Autodesk Inventor part; units mm, degrees
(part 2 of 2)
  line L438 (-36.1364, 2.6314) -> (-36.1459, 2.5251) construction
  line L439 (-36.1459, 2.5251) -> (-36.2475, 2.422) construction
  line L440 (-36.2475, 2.422) -> (-36.3751, 2.4459) construction
  line L441 (-36.3751, 2.4459) -> (-36.4459, 2.4614) construction
  spline S18 degree 3 poles (-38.8557, 2.1969) (-38.8572, 2.1987) (-38.8752, 2.2211) (-38.9092, 2.2645) (-38.9608, 2.3377) (-39.0083, 2.4172) (-39.0608, 2.5183) (-39.1072, 2.6209) (-39.1463, 2.7307) (-39.1715, 2.82) (-39.1895, 2.91) (-39.201, 2.9839) (-39.2117, 3.0528) (-39.2228, 3.1467) (-39.2255, 3.2598) (-39.2208, 3.3682) (-39.215, 3.4693) (-39.2042, 3.5799) (-39.184, 3.7003) (-39.135, 3.8891) (-39.034, 4.1141) (-38.8742, 4.3089) (-38.7335, 4.4249) (-38.62, 4.4967) (-38.5019, 4.5521) (-38.3842, 4.5944) (-38.2605, 4.6297) (-38.1226, 4.6549) (-37.9886, 4.6632) (-37.8833, 4.6627) (-37.7903, 4.6606) (-37.6909, 4.6547) (-37.5837, 4.6412) (-37.4418, 4.6164) (-37.3105, 4.5895) (-37.1813, 4.5608) (-37.0882, 4.538) (-36.9992, 4.5129) (-36.8769, 4.476) (-36.7073, 4.4231) (-36.5, 4.351) (-36.3059, 4.2743) (-36.1511, 4.2074) (-36.0218, 4.1447) (-35.903, 4.0832) (-35.7462, 3.9967) (-35.5515, 3.8647) (-35.3733, 3.7141) (-35.2209, 3.5517) (-35.1421, 3.4422) (-35.1062, 3.3821) knots 0 0 0 0 0.001093 0.013473 0.025854 0.039399 0.052944 0.078386 0.091133 0.103881 0.117308 0.130735 0.141579 0.152424 0.170959 0.189495 0.205461 0.221427 0.240479 0.259531 0.305769 0.343024 0.361055 0.379086 0.396915 0.414744 0.434745 0.454745 0.473468 0.492192 0.505844 0.519497 0.537166 0.554835 0.590157 0.606148 0.622138 0.636609 0.651081 0.687747 0.728505 0.761398 0.793268 0.812623 0.831977 0.860868 0.899522 0.942063 0.970647 1 1 1 1
  line L442 (-38.8557, 2.1969) -> (-38.8572, 2.1987) construction
  line L443 (-38.8572, 2.1987) -> (-38.8752, 2.2211) construction
  line L444 (-38.8752, 2.2211) -> (-38.9092, 2.2645) construction
  line L445 (-38.9092, 2.2645) -> (-38.9608, 2.3377) construction
  line L446 (-38.9608, 2.3377) -> (-39.0083, 2.4172) construction
  line L447 (-39.0083, 2.4172) -> (-39.0608, 2.5183) construction
  line L448 (-39.0608, 2.5183) -> (-39.1072, 2.6209) construction
  line L449 (-39.1072, 2.6209) -> (-39.1463, 2.7307) construction
  line L450 (-39.1463, 2.7307) -> (-39.1715, 2.82) construction
  line L451 (-39.1715, 2.82) -> (-39.1895, 2.91) construction
  line L452 (-39.1895, 2.91) -> (-39.201, 2.9839) construction
  line L453 (-39.201, 2.9839) -> (-39.2117, 3.0528) construction
  line L454 (-39.2117, 3.0528) -> (-39.2228, 3.1467) construction
  line L455 (-39.2228, 3.1467) -> (-39.2255, 3.2598) construction
  line L456 (-39.2255, 3.2598) -> (-39.2208, 3.3682) construction
  line L457 (-39.2208, 3.3682) -> (-39.215, 3.4693) construction
  line L458 (-39.215, 3.4693) -> (-39.2042, 3.5799) construction
  line L459 (-39.2042, 3.5799) -> (-39.184, 3.7003) construction
  line L460 (-39.184, 3.7003) -> (-39.135, 3.8891) construction
  line L461 (-39.135, 3.8891) -> (-39.034, 4.1141) construction
  line L462 (-39.034, 4.1141) -> (-38.8742, 4.3089) construction
  line L463 (-38.8742, 4.3089) -> (-38.7335, 4.4249) construction
  line L464 (-38.7335, 4.4249) -> (-38.62, 4.4967) construction
  line L465 (-38.62, 4.4967) -> (-38.5019, 4.5521) construction
  line L466 (-38.5019, 4.5521) -> (-38.3842, 4.5944) construction
  line L467 (-38.3842, 4.5944) -> (-38.2605, 4.6297) construction
  line L468 (-38.2605, 4.6297) -> (-38.1226, 4.6549) construction
  line L469 (-38.1226, 4.6549) -> (-37.9886, 4.6632) construction
  line L470 (-37.9886, 4.6632) -> (-37.8833, 4.6627) construction
  line L471 (-37.8833, 4.6627) -> (-37.7903, 4.6606) construction
  line L472 (-37.7903, 4.6606) -> (-37.6909, 4.6547) construction
  line L473 (-37.6909, 4.6547) -> (-37.5837, 4.6412) construction
  line L474 (-37.5837, 4.6412) -> (-37.4418, 4.6164) construction
  line L475 (-37.4418, 4.6164) -> (-37.3105, 4.5895) construction
  line L476 (-37.3105, 4.5895) -> (-37.1813, 4.5608) construction
  line L477 (-37.1813, 4.5608) -> (-37.0882, 4.538) construction
  line L478 (-37.0882, 4.538) -> (-36.9992, 4.5129) construction
  line L479 (-36.9992, 4.5129) -> (-36.8769, 4.476) construction
  line L480 (-36.8769, 4.476) -> (-36.7073, 4.4231) construction
  line L481 (-36.7073, 4.4231) -> (-36.5, 4.351) construction
  line L482 (-36.5, 4.351) -> (-36.3059, 4.2743) construction
  line L483 (-36.3059, 4.2743) -> (-36.1511, 4.2074) construction
  line L484 (-36.1511, 4.2074) -> (-36.0218, 4.1447) construction
  line L485 (-36.0218, 4.1447) -> (-35.903, 4.0832) construction
  line L486 (-35.903, 4.0832) -> (-35.7462, 3.9967) construction
  line L487 (-35.7462, 3.9967) -> (-35.5515, 3.8647) construction
  line L488 (-35.5515, 3.8647) -> (-35.3733, 3.7141) construction
  line L489 (-35.3733, 3.7141) -> (-35.2209, 3.5517) construction
  line L490 (-35.2209, 3.5517) -> (-35.1421, 3.4422) construction
  line L491 (-35.1421, 3.4422) -> (-35.1062, 3.3821) construction
  spline S19 degree 3 poles (-35.3209, 3.254) (-35.3774, 3.3487) (-35.5015, 3.4947) (-35.7033, 3.6655) (-35.8763, 3.7828) (-36.0526, 3.8802) (-36.221, 3.9652) (-36.4011, 4.0431) (-36.5871, 4.1166) (-36.7846, 4.1853) (-36.9771, 4.2453) (-37.1543, 4.2983) (-37.3323, 4.3387) (-37.5228, 4.3778) (-37.7065, 4.4078) (-37.8961, 4.4137) (-38.0956, 4.4123) (-38.3052, 4.3609) (-38.5029, 4.2823) (-38.6723, 4.1597) (-38.8176, 3.9829) (-38.9138, 3.7703) (-38.9587, 3.5534) (-38.9723, 3.3509) (-38.9778, 3.1783) (-38.9534, 3.0176) (-38.9313, 2.8789) (-38.8857, 2.7381) (-38.8248, 2.6032) (-38.7544, 2.4743) (-38.6401, 2.3235) (-38.5475, 2.2212) (-38.4765, 2.1644) knots 0 0 0 0 0.055351 0.095994 0.132923 0.160524 0.197506 0.227953 0.259379 0.298318 0.333348 0.360999 0.391552 0.425298 0.459059 0.485146 0.520921 0.559137 0.593204 0.627656 0.663248 0.707423 0.743827 0.774334 0.80975 0.830472 0.856127 0.880484 0.904791 0.930672 0.954328 1 1 1 1
  line L492 (-35.3209, 3.254) -> (-35.3774, 3.3487) construction
  line L493 (-35.3774, 3.3487) -> (-35.5015, 3.4947) construction
  line L494 (-35.5015, 3.4947) -> (-35.7033, 3.6655) construction
  line L495 (-35.7033, 3.6655) -> (-35.8763, 3.7828) construction
  line L496 (-35.8763, 3.7828) -> (-36.0526, 3.8802) construction
  line L497 (-36.0526, 3.8802) -> (-36.221, 3.9652) construction
  line L498 (-36.221, 3.9652) -> (-36.4011, 4.0431) construction
  line L499 (-36.4011, 4.0431) -> (-36.5871, 4.1166) construction
  line L500 (-36.5871, 4.1166) -> (-36.7846, 4.1853) construction
  line L501 (-36.7846, 4.1853) -> (-36.9771, 4.2453) construction
  line L502 (-36.9771, 4.2453) -> (-37.1543, 4.2983) construction
  line L503 (-37.1543, 4.2983) -> (-37.3323, 4.3387) construction
  line L504 (-37.3323, 4.3387) -> (-37.5228, 4.3778) construction
  line L505 (-37.5228, 4.3778) -> (-37.7065, 4.4078) construction
  line L506 (-37.7065, 4.4078) -> (-37.8961, 4.4137) construction
  line L507 (-37.8961, 4.4137) -> (-38.0956, 4.4123) construction
  line L508 (-38.0956, 4.4123) -> (-38.3052, 4.3609) construction
  line L509 (-38.3052, 4.3609) -> (-38.5029, 4.2823) construction
  line L510 (-38.5029, 4.2823) -> (-38.6723, 4.1597) construction
  line L511 (-38.6723, 4.1597) -> (-38.8176, 3.9829) construction
  line L512 (-38.8176, 3.9829) -> (-38.9138, 3.7703) construction
  line L513 (-38.9138, 3.7703) -> (-38.9587, 3.5534) construction
  line L514 (-38.9587, 3.5534) -> (-38.9723, 3.3509) construction
  line L515 (-38.9723, 3.3509) -> (-38.9778, 3.1783) construction
  line L516 (-38.9778, 3.1783) -> (-38.9534, 3.0176) construction
  line L517 (-38.9534, 3.0176) -> (-38.9313, 2.8789) construction
  line L518 (-38.9313, 2.8789) -> (-38.8857, 2.7381) construction
  line L519 (-38.8857, 2.7381) -> (-38.8248, 2.6032) construction
  line L520 (-38.8248, 2.6032) -> (-38.7544, 2.4743) construction
  line L521 (-38.7544, 2.4743) -> (-38.6401, 2.3235) construction
  line L522 (-38.6401, 2.3235) -> (-38.5475, 2.2212) construction
  line L523 (-38.5475, 2.2212) -> (-38.4765, 2.1644) construction
  spline S20 degree 3 poles (-35.1062, 3.3821) (-35.0856, 3.3476) (-35.0436, 3.2753) (-34.9846, 3.1561) (-34.9385, 3.0325) (-34.8891, 2.8556) (-34.8509, 2.5961) (-34.8504, 2.2727) (-34.9129, 1.9367) (-35.0543, 1.6251) (-35.2047, 1.4458) (-35.3027, 1.3649) knots 0 0 0 0 0.062149 0.124299 0.18074 0.237181 0.376996 0.554667 0.704453 0.841631 1 1 1 1
  line L524 (-35.1062, 3.3821) -> (-35.0856, 3.3476) construction
  line L525 (-35.0856, 3.3476) -> (-35.0436, 3.2753) construction
  line L526 (-35.0436, 3.2753) -> (-34.9846, 3.1561) construction
  line L527 (-34.9846, 3.1561) -> (-34.9385, 3.0325) construction
  line L528 (-34.9385, 3.0325) -> (-34.8891, 2.8556) construction
  line L529 (-34.8891, 2.8556) -> (-34.8509, 2.5961) construction
  line L530 (-34.8509, 2.5961) -> (-34.8504, 2.2727) construction
  line L531 (-34.8504, 2.2727) -> (-34.9129, 1.9367) construction
  line L532 (-34.9129, 1.9367) -> (-35.0543, 1.6251) construction
  line L533 (-35.0543, 1.6251) -> (-35.2047, 1.4458) construction
  line L534 (-35.2047, 1.4458) -> (-35.3027, 1.3649) construction
  spline S21 degree 3 poles (-35.7186, 1.4187) (-35.5281, 1.4749) (-35.3089, 1.6711) (-35.1543, 2.0105) (-35.1011, 2.292) (-35.1012, 2.5793) (-35.14, 2.8406) (-35.2106, 3.0616) (-35.282, 3.1887) (-35.3209, 3.254) knots 0 0 0 0 0.273796 0.392161 0.521403 0.674708 0.795348 0.892748 1 1 1 1
  line L535 (-35.7186, 1.4187) -> (-35.5281, 1.4749) construction
  line L536 (-35.5281, 1.4749) -> (-35.3089, 1.6711) construction
  line L537 (-35.3089, 1.6711) -> (-35.1543, 2.0105) construction
  line L538 (-35.1543, 2.0105) -> (-35.1011, 2.292) construction
  line L539 (-35.1011, 2.292) -> (-35.1012, 2.5793) construction
  line L540 (-35.1012, 2.5793) -> (-35.14, 2.8406) construction
  line L541 (-35.14, 2.8406) -> (-35.2106, 3.0616) construction
  line L542 (-35.2106, 3.0616) -> (-35.282, 3.1887) construction
  line L543 (-35.282, 3.1887) -> (-35.3209, 3.254) construction
  spline S22 degree 3 poles (-35.1034, -2.5702) (-35.1001, -2.5752) (-35.0478, -2.6552) (-34.986, -2.7822) (-34.9281, -2.9499) (-34.8921, -3.0945) (-34.8696, -3.2455) (-34.8592, -3.3899) (-34.856, -3.5301) (-34.8648, -3.6828) (-34.895, -3.8447) (-34.9467, -4.0029) (-35.0178, -4.1531) (-35.1217, -4.3066) (-35.267, -4.4488) (-35.4359, -4.552) (-35.598, -4.6097) (-35.7882, -4.649) (-36.0245, -4.6565) (-36.338, -4.6162) (-36.6524, -4.5374) (-36.8714, -4.4666) (-36.9719, -4.4336) knots 0 0 0 0 0.00444 0.070664 0.108166 0.145668 0.1883 0.230932 0.268421 0.305909 0.348993 0.392077 0.432213 0.472349 0.522082 0.571814 0.60605 0.640285 0.714979 0.789672 0.901222 1 1 1 1
  line L544 (-35.1034, -2.5702) -> (-35.1001, -2.5752) construction
  line L545 (-35.1001, -2.5752) -> (-35.0478, -2.6552) construction
  line L546 (-35.0478, -2.6552) -> (-34.986, -2.7822) construction
  line L547 (-34.986, -2.7822) -> (-34.9281, -2.9499) construction
  line L548 (-34.9281, -2.9499) -> (-34.8921, -3.0945) construction
  line L549 (-34.8921, -3.0945) -> (-34.8696, -3.2455) construction
  line L550 (-34.8696, -3.2455) -> (-34.8592, -3.3899) construction
  line L551 (-34.8592, -3.3899) -> (-34.856, -3.5301) construction
  line L552 (-34.856, -3.5301) -> (-34.8648, -3.6828) construction
  line L553 (-34.8648, -3.6828) -> (-34.895, -3.8447) construction
  line L554 (-34.895, -3.8447) -> (-34.9467, -4.0029) construction
  line L555 (-34.9467, -4.0029) -> (-35.0178, -4.1531) construction
  line L556 (-35.0178, -4.1531) -> (-35.1217, -4.3066) construction
  line L557 (-35.1217, -4.3066) -> (-35.267, -4.4488) construction
  line L558 (-35.267, -4.4488) -> (-35.4359, -4.552) construction
  line L559 (-35.4359, -4.552) -> (-35.598, -4.6097) construction
  line L560 (-35.598, -4.6097) -> (-35.7882, -4.649) construction
  line L561 (-35.7882, -4.649) -> (-36.0245, -4.6565) construction
  line L562 (-36.0245, -4.6565) -> (-36.338, -4.6162) construction
  line L563 (-36.338, -4.6162) -> (-36.6524, -4.5374) construction
  line L564 (-36.6524, -4.5374) -> (-36.8714, -4.4666) construction
  line L565 (-36.8714, -4.4666) -> (-36.9719, -4.4336) construction
  spline S23 degree 3 poles (-36.9719, -4.4336) (-37.0123, -4.4203) (-37.0897, -4.3922) (-37.2189, -4.342) (-37.3714, -4.2863) (-37.5356, -4.2233) (-37.6712, -4.1641) (-37.8012, -4.1048) (-37.9577, -4.0339) (-38.1361, -3.9493) (-38.3019, -3.864) (-38.4383, -3.7917) (-38.5691, -3.7231) (-38.6924, -3.6501) (-38.8071, -3.5657) (-38.9238, -3.4587) (-39.0391, -3.3162) (-39.129, -3.1482) (-39.1807, -2.9867) (-39.2052, -2.8557) (-39.217, -2.7336) (-39.2183, -2.6183) (-39.2094, -2.5046) (-39.1927, -2.3995) (-39.1684, -2.2913) (-39.1263, -2.1755) (-39.0633, -2.0679) (-38.991, -1.9827) (-38.9362, -1.9368) (-38.9114, -1.9187) knots 0 0 0 0 0.033633 0.067267 0.12497 0.182674 0.216203 0.249732 0.309838 0.369945 0.420395 0.470846 0.5098 0.548753 0.581089 0.613424 0.660377 0.707331 0.741496 0.77566 0.80376 0.83186 0.859174 0.886489 0.912352 0.938215 0.960595 0.982975 1 1 1 1
  line L566 (-36.9719, -4.4336) -> (-37.0123, -4.4203) construction
  line L567 (-37.0123, -4.4203) -> (-37.0897, -4.3922) construction
  line L568 (-37.0897, -4.3922) -> (-37.2189, -4.342) construction
  line L569 (-37.2189, -4.342) -> (-37.3714, -4.2863) construction
  line L570 (-37.3714, -4.2863) -> (-37.5356, -4.2233) construction
  line L571 (-37.5356, -4.2233) -> (-37.6712, -4.1641) construction
  line L572 (-37.6712, -4.1641) -> (-37.8012, -4.1048) construction
  line L573 (-37.8012, -4.1048) -> (-37.9577, -4.0339) construction
  line L574 (-37.9577, -4.0339) -> (-38.1361, -3.9493) construction
  line L575 (-38.1361, -3.9493) -> (-38.3019, -3.864) construction
  line L576 (-38.3019, -3.864) -> (-38.4383, -3.7917) construction
  line L577 (-38.4383, -3.7917) -> (-38.5691, -3.7231) construction
  line L578 (-38.5691, -3.7231) -> (-38.6924, -3.6501) construction
  line L579 (-38.6924, -3.6501) -> (-38.8071, -3.5657) construction
  line L580 (-38.8071, -3.5657) -> (-38.9238, -3.4587) construction
  line L581 (-38.9238, -3.4587) -> (-39.0391, -3.3162) construction
  line L582 (-39.0391, -3.3162) -> (-39.129, -3.1482) construction
  line L583 (-39.129, -3.1482) -> (-39.1807, -2.9867) construction
  line L584 (-39.1807, -2.9867) -> (-39.2052, -2.8557) construction
  line L585 (-39.2052, -2.8557) -> (-39.217, -2.7336) construction
  line L586 (-39.217, -2.7336) -> (-39.2183, -2.6183) construction
  line L587 (-39.2183, -2.6183) -> (-39.2094, -2.5046) construction
  line L588 (-39.2094, -2.5046) -> (-39.1927, -2.3995) construction
  line L589 (-39.1927, -2.3995) -> (-39.1684, -2.2913) construction
  line L590 (-39.1684, -2.2913) -> (-39.1263, -2.1755) construction
  line L591 (-39.1263, -2.1755) -> (-39.0633, -2.0679) construction
  line L592 (-39.0633, -2.0679) -> (-38.991, -1.9827) construction
  line L593 (-38.991, -1.9827) -> (-38.9362, -1.9368) construction
  line L594 (-38.9362, -1.9368) -> (-38.9114, -1.9187) construction
  spline S24 degree 3 poles (-38.9114, -1.9187) (-38.9251, -1.9011) (-38.9697, -1.8403) (-39.0351, -1.7307) (-39.0942, -1.6025) (-39.1398, -1.4803) (-39.181, -1.3363) (-39.2151, -1.1313) (-39.2281, -0.9209) (-39.2377, -0.6906) (-39.226, -0.4881) (-39.1858, -0.3064) (-39.1385, -0.1725) (-39.0783, -0.0531) (-39.0252, 0.0316) (-38.9882, 0.0842) (-38.973, 0.104) knots 0 0 0 0 0.029625 0.099401 0.169177 0.226396 0.283615 0.373252 0.518061 0.616606 0.732557 0.796641 0.860726 0.914778 0.96883 1 1 1 1
  line L595 (-38.9114, -1.9187) -> (-38.9251, -1.9011) construction
  line L596 (-38.9251, -1.9011) -> (-38.9697, -1.8403) construction
  line L597 (-38.9697, -1.8403) -> (-39.0351, -1.7307) construction
  line L598 (-39.0351, -1.7307) -> (-39.0942, -1.6025) construction
  line L599 (-39.0942, -1.6025) -> (-39.1398, -1.4803) construction
  line L600 (-39.1398, -1.4803) -> (-39.181, -1.3363) construction
  line L601 (-39.181, -1.3363) -> (-39.2151, -1.1313) construction
  line L602 (-39.2151, -1.1313) -> (-39.2281, -0.9209) construction
  line L603 (-39.2281, -0.9209) -> (-39.2377, -0.6906) construction
  line L604 (-39.2377, -0.6906) -> (-39.226, -0.4881) construction
  line L605 (-39.226, -0.4881) -> (-39.1858, -0.3064) construction
  line L606 (-39.1858, -0.3064) -> (-39.1385, -0.1725) construction
  line L607 (-39.1385, -0.1725) -> (-39.0783, -0.0531) construction
  line L608 (-39.0783, -0.0531) -> (-39.0252, 0.0316) construction
  line L609 (-39.0252, 0.0316) -> (-38.9882, 0.0842) construction
  line L610 (-38.9882, 0.0842) -> (-38.973, 0.104) construction
  spline S25 degree 3 poles (-35.137, -0.7452) (-35.1273, -0.7589) (-35.0841, -0.8224) (-35.0167, -0.9412) (-34.9453, -1.1152) (-34.8975, -1.2995) (-34.8655, -1.5015) (-34.842, -1.7306) (-34.8544, -1.977) (-34.9084, -2.186) (-34.9802, -2.3655) (-35.0495, -2.4912) (-35.0989, -2.5638) (-35.1034, -2.5702) knots 0 0 0 0 0.025339 0.116179 0.207018 0.309076 0.411134 0.550932 0.69073 0.778469 0.866209 0.988083 1 1 1 1
  line L611 (-35.137, -0.7452) -> (-35.1273, -0.7589) construction
  line L612 (-35.1273, -0.7589) -> (-35.0841, -0.8224) construction
  line L613 (-35.0841, -0.8224) -> (-35.0167, -0.9412) construction
  line L614 (-35.0167, -0.9412) -> (-34.9453, -1.1152) construction
  line L615 (-34.9453, -1.1152) -> (-34.8975, -1.2995) construction
  line L616 (-34.8975, -1.2995) -> (-34.8655, -1.5015) construction
  line L617 (-34.8655, -1.5015) -> (-34.842, -1.7306) construction
  line L618 (-34.842, -1.7306) -> (-34.8544, -1.977) construction
  line L619 (-34.8544, -1.977) -> (-34.9084, -2.186) construction
  line L620 (-34.9084, -2.186) -> (-34.9802, -2.3655) construction
  line L621 (-34.9802, -2.3655) -> (-35.0495, -2.4912) construction
  line L622 (-35.0495, -2.4912) -> (-35.0989, -2.5638) construction
  line L623 (-35.0989, -2.5638) -> (-35.1034, -2.5702) construction
  arc A2 (-37.8544, -1.1308) -> (-37.4616, -1.3224) centre (-36.4977, 1.1532) ccw
  arc A3 (-36.7641, -1.5741) -> (-36.2828, -1.7225) centre (-35.1742, 2.7263) ccw
  spline S26 degree 3 poles (-36.7641, -1.5741) (-36.7505, -1.4891) (-36.7247, -1.3264) (-36.7301, -1.0707) (-36.8177, -0.8355) (-37.0007, -0.7186) (-37.1591, -0.6557) (-37.3343, -0.6531) (-37.4608, -0.8025) (-37.4863, -1.0375) (-37.4849, -1.2137) (-37.4616, -1.3224) knots 0.000002 0.000002 0.000002 0.000002 0.130512 0.248338 0.387441 0.486956 0.566128 0.647917 0.731171 0.833817 0.999993 0.999993 0.999993 0.999993
  line L624 (-36.7641, -1.5741) -> (-36.7505, -1.4891) construction
  line L625 (-36.7505, -1.4891) -> (-36.7247, -1.3264) construction
  line L626 (-36.7247, -1.3264) -> (-36.7301, -1.0707) construction
  line L627 (-36.7301, -1.0707) -> (-36.8177, -0.8355) construction
  line L628 (-36.8177, -0.8355) -> (-37.0007, -0.7186) construction
  line L629 (-37.0007, -0.7186) -> (-37.1591, -0.6557) construction
  line L630 (-37.1591, -0.6557) -> (-37.3343, -0.6531) construction
  line L631 (-37.3343, -0.6531) -> (-37.4608, -0.8025) construction
  line L632 (-37.4608, -0.8025) -> (-37.4863, -1.0375) construction
  line L633 (-37.4863, -1.0375) -> (-37.4849, -1.2137) construction
  line L634 (-37.4849, -1.2137) -> (-37.4616, -1.3224) construction
  spline S27 degree 3 poles (-35.4263, -2.5707) (-35.3321, -2.4741) (-35.2054, -2.2811) (-35.0814, -1.9154) (-35.1051, -1.552) (-35.1862, -1.1164) (-35.3442, -0.8602) (-35.473, -0.7347) knots 0 0 0 0 0.199784 0.341442 0.567149 0.731925 1 1 1 1
  line L635 (-35.4263, -2.5707) -> (-35.3321, -2.4741) construction
  line L636 (-35.3321, -2.4741) -> (-35.2054, -2.2811) construction
  line L637 (-35.2054, -2.2811) -> (-35.0814, -1.9154) construction
  line L638 (-35.0814, -1.9154) -> (-35.1051, -1.552) construction
  line L639 (-35.1051, -1.552) -> (-35.1862, -1.1164) construction
  line L640 (-35.1862, -1.1164) -> (-35.3442, -0.8602) construction
  line L641 (-35.3442, -0.8602) -> (-35.473, -0.7347) construction
  spline S28 degree 3 poles (-37.8544, -1.1308) (-37.8536, -0.9801) (-37.8499, -0.742) (-37.9125, -0.4332) (-38.0504, -0.2331) (-38.2518, -0.153) (-38.4786, -0.1595) (-38.6195, -0.3388) (-38.6813, -0.5514) (-38.6938, -0.7925) (-38.677, -1.0533) (-38.6261, -1.3179) (-38.5012, -1.5537) (-38.3084, -1.7405) (-38.0832, -1.8914) (-37.839, -2.0089) (-37.5863, -2.1154) (-37.3337, -2.2319) (-37.0665, -2.3111) (-36.8068, -2.3986) (-36.5292, -2.458) (-36.2438, -2.5065) (-35.9696, -2.5082) (-35.7113, -2.4196) (-35.5214, -2.2369) (-35.4217, -1.9412) (-35.3888, -1.645) (-35.4563, -1.3237) (-35.5661, -1.0472) (-35.7908, -0.8404) (-36.0487, -0.7938) (-36.2934, -0.8932) (-36.3899, -1.2666) (-36.3184, -1.5315) (-36.2828, -1.7225) knots 0.000002 0.000002 0.000002 0.000002 0.050812 0.079978 0.105051 0.128715 0.150613 0.176165 0.198359 0.225349 0.256757 0.286428 0.315385 0.345015 0.375912 0.406383 0.43613 0.468337 0.499902 0.529857 0.5606 0.595385 0.627424 0.651669 0.685878 0.711437 0.755573 0.784369 0.821416 0.854265 0.882212 0.905839 0.935385 1 1 1 1
  line L642 (-37.8544, -1.1308) -> (-37.8536, -0.9801) construction
  line L643 (-37.8536, -0.9801) -> (-37.8499, -0.742) construction
  line L644 (-37.8499, -0.742) -> (-37.9125, -0.4332) construction
  line L645 (-37.9125, -0.4332) -> (-38.0504, -0.2331) construction
  line L646 (-38.0504, -0.2331) -> (-38.2518, -0.153) construction
  line L647 (-38.2518, -0.153) -> (-38.4786, -0.1595) construction
  line L648 (-38.4786, -0.1595) -> (-38.6195, -0.3388) construction
  line L649 (-38.6195, -0.3388) -> (-38.6813, -0.5514) construction
  line L650 (-38.6813, -0.5514) -> (-38.6938, -0.7925) construction
  line L651 (-38.6938, -0.7925) -> (-38.677, -1.0533) construction
  line L652 (-38.677, -1.0533) -> (-38.6261, -1.3179) construction
  line L653 (-38.6261, -1.3179) -> (-38.5012, -1.5537) construction
  line L654 (-38.5012, -1.5537) -> (-38.3084, -1.7405) construction
  line L655 (-38.3084, -1.7405) -> (-38.0832, -1.8914) construction
  line L656 (-38.0832, -1.8914) -> (-37.839, -2.0089) construction
  line L657 (-37.839, -2.0089) -> (-37.5863, -2.1154) construction
  line L658 (-37.5863, -2.1154) -> (-37.3337, -2.2319) construction
  line L659 (-37.3337, -2.2319) -> (-37.0665, -2.3111) construction
  line L660 (-37.0665, -2.3111) -> (-36.8068, -2.3986) construction
  line L661 (-36.8068, -2.3986) -> (-36.5292, -2.458) construction
  line L662 (-36.5292, -2.458) -> (-36.2438, -2.5065) construction
  line L663 (-36.2438, -2.5065) -> (-35.9696, -2.5082) construction
  line L664 (-35.9696, -2.5082) -> (-35.7113, -2.4196) construction
  line L665 (-35.7113, -2.4196) -> (-35.5214, -2.2369) construction
  line L666 (-35.5214, -2.2369) -> (-35.4217, -1.9412) construction
  line L667 (-35.4217, -1.9412) -> (-35.3888, -1.645) construction
  line L668 (-35.3888, -1.645) -> (-35.4563, -1.3237) construction
  line L669 (-35.4563, -1.3237) -> (-35.5661, -1.0472) construction
  line L670 (-35.5661, -1.0472) -> (-35.7908, -0.8404) construction
  line L671 (-35.7908, -0.8404) -> (-36.0487, -0.7938) construction
  line L672 (-36.0487, -0.7938) -> (-36.2934, -0.8932) construction
  line L673 (-36.2934, -0.8932) -> (-36.3899, -1.2666) construction
  line L674 (-36.3899, -1.2666) -> (-36.3184, -1.5315) construction
  line L675 (-36.3184, -1.5315) -> (-36.2828, -1.7225) construction
  spline S29 degree 3 poles (-36.295, -3.2208) (-36.3961, -3.1865) (-36.6076, -3.0929) (-36.9302, -2.923) (-37.2988, -2.7694) (-37.6429, -2.612) (-37.947, -2.4624) (-38.2101, -2.395) (-38.4408, -2.3351) (-38.6523, -2.4559) (-38.6702, -2.686) (-38.6453, -2.8298) (-38.6227, -2.8984) knots 0 0 0 0 0.107518 0.23411 0.368721 0.511133 0.617815 0.709418 0.788123 0.85006 0.926906 1 1 1 1
  line L676 (-36.295, -3.2208) -> (-36.3961, -3.1865) construction
  line L677 (-36.3961, -3.1865) -> (-36.6076, -3.0929) construction
  line L678 (-36.6076, -3.0929) -> (-36.9302, -2.923) construction
  line L679 (-36.9302, -2.923) -> (-37.2988, -2.7694) construction
  line L680 (-37.2988, -2.7694) -> (-37.6429, -2.612) construction
  line L681 (-37.6429, -2.612) -> (-37.947, -2.4624) construction
  line L682 (-37.947, -2.4624) -> (-38.2101, -2.395) construction
  line L683 (-38.2101, -2.395) -> (-38.4408, -2.3351) construction
  line L684 (-38.4408, -2.3351) -> (-38.6523, -2.4559) construction
  line L685 (-38.6523, -2.4559) -> (-38.6702, -2.686) construction
  line L686 (-38.6702, -2.686) -> (-38.6453, -2.8298) construction
  line L687 (-38.6453, -2.8298) -> (-38.6227, -2.8984) construction
  spline S30 degree 3 poles (-38.6227, -2.8984) (-38.5671, -3.0675) (-38.3501, -3.2221) (-38.0283, -3.3874) (-37.7632, -3.5103) (-37.4823, -3.6447) (-37.1771, -3.7647) (-36.8447, -3.8847) (-36.5182, -4.002) (-36.1996, -4.0704) (-35.8996, -4.1189) (-35.6034, -4.042) (-35.4212, -3.7695) (-35.4175, -3.442) (-35.4429, -3.1128) (-35.5754, -2.8248) (-35.7947, -2.6631) (-36.0051, -2.6098) (-36.201, -2.6189) (-36.2695, -2.7587) (-36.3466, -2.9422) (-36.295, -3.1086) (-36.295, -3.2208) knots 0 0 0 0 0.084367 0.132854 0.185682 0.233817 0.292249 0.353411 0.414803 0.469553 0.519939 0.570079 0.615873 0.676082 0.733974 0.784619 0.833154 0.866506 0.897762 0.921095 0.940031 1 1 1 1
  line L688 (-38.6227, -2.8984) -> (-38.5671, -3.0675) construction
  line L689 (-38.5671, -3.0675) -> (-38.3501, -3.2221) construction
  line L690 (-38.3501, -3.2221) -> (-38.0283, -3.3874) construction
  line L691 (-38.0283, -3.3874) -> (-37.7632, -3.5103) construction
  line L692 (-37.7632, -3.5103) -> (-37.4823, -3.6447) construction
  line L693 (-37.4823, -3.6447) -> (-37.1771, -3.7647) construction
  line L694 (-37.1771, -3.7647) -> (-36.8447, -3.8847) construction
  line L695 (-36.8447, -3.8847) -> (-36.5182, -4.002) construction
  line L696 (-36.5182, -4.002) -> (-36.1996, -4.0704) construction
  line L697 (-36.1996, -4.0704) -> (-35.8996, -4.1189) construction
  line L698 (-35.8996, -4.1189) -> (-35.6034, -4.042) construction
  line L699 (-35.6034, -4.042) -> (-35.4212, -3.7695) construction
  line L700 (-35.4212, -3.7695) -> (-35.4175, -3.442) construction
  line L701 (-35.4175, -3.442) -> (-35.4429, -3.1128) construction
  line L702 (-35.4429, -3.1128) -> (-35.5754, -2.8248) construction
  line L703 (-35.5754, -2.8248) -> (-35.7947, -2.6631) construction
  line L704 (-35.7947, -2.6631) -> (-36.0051, -2.6098) construction
  line L705 (-36.0051, -2.6098) -> (-36.201, -2.6189) construction
  line L706 (-36.201, -2.6189) -> (-36.2695, -2.7587) construction
  line L707 (-36.2695, -2.7587) -> (-36.3466, -2.9422) construction
  line L708 (-36.3466, -2.9422) -> (-36.295, -3.1086) construction
  line L709 (-36.295, -3.1086) -> (-36.295, -3.2208) construction
  spline S31 degree 3 poles (-36.894, -4.196) (-36.6814, -4.2658) (-36.3179, -4.3813) (-35.8552, -4.4183) (-35.5253, -4.3309) (-35.3092, -4.1612) (-35.1706, -3.9109) (-35.1064, -3.6593) (-35.106, -3.3965) (-35.1308, -3.1469) (-35.2179, -2.853) (-35.3276, -2.6646) (-35.4263, -2.5707) knots 0 0 0 0 0.199139 0.340579 0.405407 0.499581 0.575583 0.657166 0.728155 0.808883 0.879897 1 1 1 1
  line L710 (-36.894, -4.196) -> (-36.6814, -4.2658) construction
  line L711 (-36.6814, -4.2658) -> (-36.3179, -4.3813) construction
  line L712 (-36.3179, -4.3813) -> (-35.8552, -4.4183) construction
  line L713 (-35.8552, -4.4183) -> (-35.5253, -4.3309) construction
  line L714 (-35.5253, -4.3309) -> (-35.3092, -4.1612) construction
  line L715 (-35.3092, -4.1612) -> (-35.1706, -3.9109) construction
  line L716 (-35.1706, -3.9109) -> (-35.1064, -3.6593) construction
  line L717 (-35.1064, -3.6593) -> (-35.106, -3.3965) construction
  line L718 (-35.106, -3.3965) -> (-35.1308, -3.1469) construction
  line L719 (-35.1308, -3.1469) -> (-35.2179, -2.853) construction
  line L720 (-35.2179, -2.853) -> (-35.3276, -2.6646) construction
  line L721 (-35.3276, -2.6646) -> (-35.4263, -2.5707) construction
  spline S32 degree 3 poles (-38.4224, -2.0305) (-38.511, -2.0285) (-38.6544, -2.0444) (-38.8148, -2.1513) (-38.9068, -2.2823) (-38.9502, -2.4471) (-38.9722, -2.6273) (-38.9611, -2.8276) (-38.9038, -3.0668) (-38.7584, -3.2827) (-38.5523, -3.4497) (-38.3111, -3.5758) (-38.0172, -3.7325) (-37.7244, -3.865) (-37.4173, -4.005) (-37.1546, -4.0976) (-36.9652, -4.1726) (-36.894, -4.196) knots 0 0 0 0 0.072614 0.112271 0.152694 0.199409 0.248745 0.299499 0.361207 0.446015 0.504419 0.574777 0.665902 0.774466 0.835026 0.939251 1 1 1 1
  line L722 (-38.4224, -2.0305) -> (-38.511, -2.0285) construction
  line L723 (-38.511, -2.0285) -> (-38.6544, -2.0444) construction
  line L724 (-38.6544, -2.0444) -> (-38.8148, -2.1513) construction
  line L725 (-38.8148, -2.1513) -> (-38.9068, -2.2823) construction
  line L726 (-38.9068, -2.2823) -> (-38.9502, -2.4471) construction
  line L727 (-38.9502, -2.4471) -> (-38.9722, -2.6273) construction
  line L728 (-38.9722, -2.6273) -> (-38.9611, -2.8276) construction
  line L729 (-38.9611, -2.8276) -> (-38.9038, -3.0668) construction
  line L730 (-38.9038, -3.0668) -> (-38.7584, -3.2827) construction
  line L731 (-38.7584, -3.2827) -> (-38.5523, -3.4497) construction
  line L732 (-38.5523, -3.4497) -> (-38.3111, -3.5758) construction
  line L733 (-38.3111, -3.5758) -> (-38.0172, -3.7325) construction
  line L734 (-38.0172, -3.7325) -> (-37.7244, -3.865) construction
  line L735 (-37.7244, -3.865) -> (-37.4173, -4.005) construction
  line L736 (-37.4173, -4.005) -> (-37.1546, -4.0976) construction
  line L737 (-37.1546, -4.0976) -> (-36.9652, -4.1726) construction
  line L738 (-36.9652, -4.1726) -> (-36.894, -4.196) construction
  spline S33 degree 3 poles (-38.6415, 0.0726) (-38.6724, 0.0558) (-38.7345, 0.0067) (-38.8221, -0.1099) (-38.9162, -0.2732) (-38.9746, -0.4812) (-38.9873, -0.6891) (-38.9786, -0.9065) (-38.9657, -1.1079) (-38.9305, -1.3167) (-38.8644, -1.5148) (-38.7682, -1.7022) (-38.6184, -1.8835) (-38.5031, -1.9808) (-38.4224, -2.0305) knots 0 0 0 0 0.043128 0.099176 0.181255 0.278569 0.366606 0.441427 0.551375 0.619433 0.706321 0.812277 0.88131 1 1 1 1
  line L739 (-38.6415, 0.0726) -> (-38.6724, 0.0558) construction
  line L740 (-38.6724, 0.0558) -> (-38.7345, 0.0067) construction
  line L741 (-38.7345, 0.0067) -> (-38.8221, -0.1099) construction
  line L742 (-38.8221, -0.1099) -> (-38.9162, -0.2732) construction
  line L743 (-38.9162, -0.2732) -> (-38.9746, -0.4812) construction
  line L744 (-38.9746, -0.4812) -> (-38.9873, -0.6891) construction
  line L745 (-38.9873, -0.6891) -> (-38.9786, -0.9065) construction
  line L746 (-38.9786, -0.9065) -> (-38.9657, -1.1079) construction
  line L747 (-38.9657, -1.1079) -> (-38.9305, -1.3167) construction
  line L748 (-38.9305, -1.3167) -> (-38.8644, -1.5148) construction
  line L749 (-38.8644, -1.5148) -> (-38.7682, -1.7022) construction
  line L750 (-38.7682, -1.7022) -> (-38.6184, -1.8835) construction
  line L751 (-38.6184, -1.8835) -> (-38.5031, -1.9808) construction
  line L752 (-38.5031, -1.9808) -> (-38.4224, -2.0305) construction
  line L753 (-43.5, 12.4876) -> (-43.5, -12.4876) projected
  point P0 (0, 0)
  point P1 (-43.5, 0)
  point P2 (-37.3738, 4.0435)
  point P3 (-36.5672, 0.7572)
  point P4 (-36.653, 0.7791)
  point P5 (-37.8544, -1.1308)
  point P6 (-36.2828, -1.7225)
  point P7 (-37.4616, -1.3224)
  point P8 (-35.1062, 3.3821)
  point P9 (-38.9753, 0.1076)
  point P10 (-38.9164, -1.9122)
  point P11 (-36.9727, -4.4333)
  point P12 (-35.137, -0.7452)
  point P13 (-35.4728, -0.7345)
  point P14 (-35.4239, -2.5731)
  point P15 (-38.4237, -2.0297)
  point P16 (-38.6415, 0.0726)
  point P17 (-38.477, 2.1642)
  point P18 (-35.3209, 3.254)
  point P19 (-35.7117, 1.4133)
  point P20 (-32.0833, -4.9167)
  dimension "d51" = 1.5
  dimension "d52" = 5
  constraints: 20 end point, 8 point on circle, 4 centre point, 1 midpoint, 99 other
  measures "d51" distance from line of point (-42, -5) L753
  measures "d52" vertical distance of point (-43.5, 0) point (-42, -5)
extrude "Extrusion8" cut sketch "Skizze8" against normal blind 0.1
equation "\"d9\" = d10"
equation "\"d15\" = d10"
equation "\"d47\" = d46"
equation "\"d43\" = d42"
